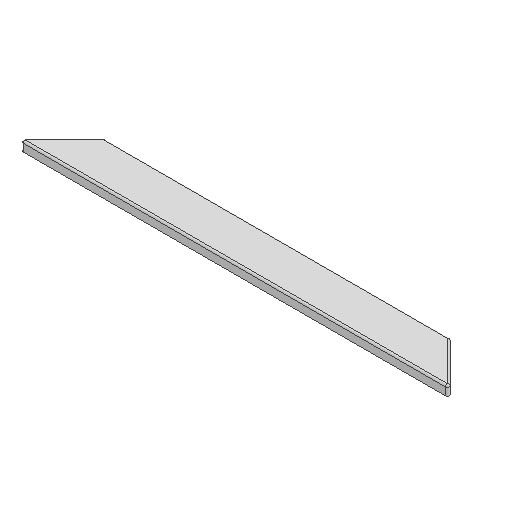
# Autodesk Inventor part: Border
Saved by Autodesk Inventor 2025.2 (Build 292293000, 293)
## iProperties
Created: 2025-03-03
Part Number: Border
Material: Generic
Document SubType Name: Modeling
Designer: Marcu
Density: 1 g/cm^3
Appearance: Default
Author: Marcu
Autodesk Inventor part; units mm, degrees
ref_plane "YZ Plane" through (0, 0, 0) normal (1, 0, 0) x (0, 1, 0)
ref_plane "XZ Plane" through (0, 0, 0) normal (0, 1, 0) x (-1, 0, 0)
ref_plane "XY Plane" through (0, 0, 0) normal (0, 0, 1) x (1, 0, 0)
sketch "Sketch1" plane through (0, 0, 0) normal (0, 0, 1) x (1, 0, 0)
  line L0 (-180, 0) -> (180, 0)
  line L1 (-225, -45) -> (225, -45)
  line L2 (-180, 0) -> (-225, -45)
  line L3 (180, 0) -> (225, -45)
  point P0 (0, 0)
  point P1 (0, 0)
  dimension "d0" = 360
  dimension "d1" = 180
  dimension "d2" = 45
  dimension "d3" = 450
  dimension "d4" = 225
  constraints: 8 end point, 1 horizontal, 1 midpoint, 1 parallel
  measures "d0" distance of L0.start L0.end
  measures "d1" distance of point (0, 0) L0.start
  measures "d2" distance between parallel lines of L0 L1
  measures "d3" distance of L1.end L1.start
  measures "d4" horizontal distance of point (0, 0) L1.end
extrude "Extrusion1" add sketch "Sketch1" along normal blind 10
fillet "Fillet1" radius 2 4 edges at (225, -45, 5) (180, 0, 5) (-180, 0, 5) (-225, -45, 5)
fillet "Fillet2" radius 2 8 edges at (222.0193, -43.7654, 10) (201.0858, -21.0858, 10) (179.9369, -0.1522, 10) (0, 0, 10) (-179.9369, -0.1522, 10) (-201.0858, -21.0858, 10) (-222.0193, -43.7654, 10) (0, -45, 10)
body "Solid1"
